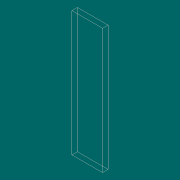
# Autodesk Inventor part: A1-18002-100-53 Tube stop
Saved by Autodesk Inventor 2017 (Build 210142000, 142)
## iProperties
Created: 2018-06-13
Part Number: A1-18002-100-53 Tube stop
Material: Steel, Mild
Document SubType Name: Modeling
Designer: Graeme_Van_Dongen
Density: 7.85 g/cm^3
Appearance: Steel
Author: Graeme_Van_Dongen
Autodesk Inventor part; units mm, degrees
ref_plane "YZ Plane" through (0, 0, 0) normal (1, 0, 0) x (0, 1, 0)
ref_plane "XZ Plane" through (0, 0, 0) normal (0, 1, 0) x (-1, 0, 0)
ref_plane "XY Plane" through (0, 0, 0) normal (0, 0, 1) x (1, 0, 0)
sketch "Sketch1" plane through (0, 0, 0) normal (0, 0, 1) x (1, 0, 0)
  line L0 (0, 0) -> (17.1196, 0)
  line L1 (17.1196, 0) -> (17.1196, 69.85)
  line L2 (17.1196, 69.85) -> (0, 69.85)
  line L3 (0, 69.85) -> (0, 0)
  dimension "d0" = 17.1196
  dimension "d1" = 69.85
  constraints: 8 end point, 2 parallel, 1 horizontal, 1 perpendicular
  measures "d0" distance of L2.end L1.end
  measures "d1" distance of L1.end L0.end
extrude "Extrusion1" add sketch "Sketch1" along normal mid plane 3.048
body "Solid1"
